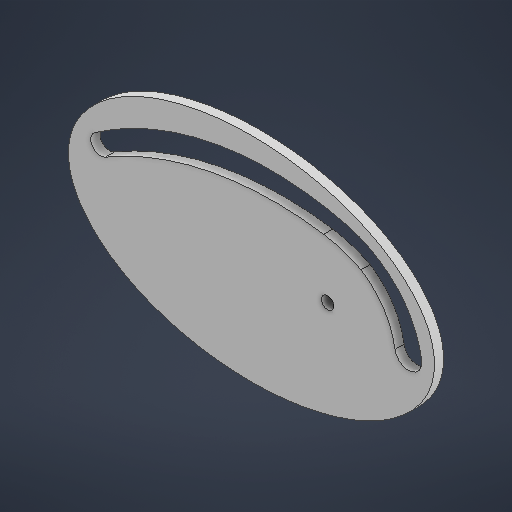
# Autodesk Inventor part: Rail1st_withoutD
Saved by Autodesk Inventor 2027 (Build 310192000, 192)
## iProperties
Created: 2026-05-09
Part Number: Rail1st_withoutD
Material: Generic
Document SubType Name: Modeling
Designer: alexy
Density: 1 g/cm^3
Appearance: Default
Author: alexy
Autodesk Inventor part; units mm, degrees
ref_plane "YZ Plane" through (0, 0, 0) normal (1, 0, 0) x (0, 1, 0)
ref_plane "XZ Plane" through (0, 0, 0) normal (0, 1, 0) x (-1, 0, 0)
ref_plane "XY Plane" through (0, 0, 0) normal (0, 0, 1) x (1, 0, 0)
sketch "Sketch1" plane through (0, 0, 0) normal (0, 0, 1) x (1, 0, 0)
  ellipse E0 centre (0, 0) end of major axis (60, 0) minor radius 35
  arc A0 (31.7478, 25.0725) -> (-51.1828, 10.244) centre (6.3686, -72.3059) ccw
  arc A1 (23.7013, 18.7616) -> (-47.9094, 4.8665) centre (7.508, -89.26) ccw
  arc A2 (55.8771, -1.3072) -> (42.2522, 20.2317) centre (25.552, -5.4112) ccw
  arc A3 (47.0757, -2.2311) -> (35.9428, 14.8131) centre (22.8888, -5.8715) ccw
  arc A4 (35.9428, 14.8131) -> (23.7013, 18.7616) centre (17.8337, -20.3799) ccw
  arc A5 (42.2522, 20.2317) -> (31.7478, 25.0725) centre (23.4586, -6.7326) ccw
  arc A6 (-51.1828, 10.244) -> (-47.9094, 4.8665) centre (-49.5461, 7.5553) ccw
  arc A7 (47.0757, -2.2311) -> (55.8771, -1.3072) centre (51.4557, -1.5719) ccw
  circle A8 centre (25, 0) radius 2.05
  dimension "d0" = 60
  dimension "d1" = 35
  dimension "d7" = 4.1
  dimension "d8" = 25
  constraints: 17 point on circle, 10 centre point, 3 tangent, 1 coincident, 1 horizontal alignment, 1 other
  measures "d7" diameter of A8
  measures "d8" distance of point (0, 0) A8.centre
extrude "Extrusion1" add sketch "Sketch1" along normal blind 3
body "Solid1"
